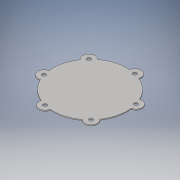
# Autodesk Inventor part: Base_bottom
Saved by Autodesk Inventor 2016 (Build 200138000, 138)
## iProperties
Created: 2015-10-08
Part Number: Base_bottom
Material: Generic
Document SubType Name: Modeling
Designer: powasar16
Density: 1 g/cm^3
Appearance: Default
Author: powasar16
Autodesk Inventor part; units mm, degrees
ref_plane "YZ Plane" through (0, 0, 0) normal (1, 0, 0) x (0, 1, 0)
ref_plane "XZ Plane" through (0, 0, 0) normal (0, 1, 0) x (-1, 0, 0)
ref_plane "XY Plane" through (0, 0, 0) normal (0, 0, 1) x (1, 0, 0)
sketch "Sketch1" plane through (0, 0, 0) normal (0, 1, 0) x (-1, 0, 0)
  circle A0 centre (54.9831, -52.757) radius 12.7
  circle A1 centre (73.1804, 21.2382) radius 12.7
  circle A2 centre (18.1974, 73.9952) radius 12.7
  circle A3 centre (-54.9831, 52.757) radius 12.7
  circle A4 centre (-73.1804, -21.2382) radius 12.7
  circle A5 centre (-18.1974, -73.9952) radius 12.7
  circle A6 centre (54.9831, -52.757) radius 3.75
  circle A7 centre (73.1804, 21.2382) radius 3.75
  circle A8 centre (18.1974, 73.9952) radius 3.75
  circle A9 centre (-54.9831, 52.757) radius 3.75
  circle A10 centre (-73.1804, -21.2382) radius 3.75
  circle A11 centre (-18.1974, -73.9952) radius 3.75
  arc A12 (72.047, 24.8128) -> (21.8158, 73.0104) centre (0, 0) ccw
  arc A13 (57.512, -49.9881) -> (74.1367, 17.6122) centre (0, 0) ccw
  arc A14 (-14.535, -74.8009) -> (52.321, -55.3982) centre (0, 0) ccw
  arc A15 (-72.047, -24.8128) -> (-21.8158, -73.0104) centre (0, 0) ccw
  arc A16 (14.535, 74.8009) -> (-52.321, 55.3982) centre (0, 0) ccw
  arc A17 (-57.512, 49.9881) -> (-74.1367, -17.6122) centre (0, 0) ccw
  point P0 (73.9952, -18.1974)
  dimension "d7" = 25.4
  dimension "d12" = 360
  dimension "d15" = 7.5
  dimension "d18" = 360
  constraints: 25 point on circle, 18 centre point, 2 coincident, 32 other
  measures "d7" diameter of A0
  measures "d15" diameter of A6
extrude "Extrusion1" add sketch "Sketch1" along normal blind 1.905 contours A0 A14 A6 A13 | A13 A6 A14 A0 | A0 A14 A5 A15 A4 A17 A3 A16 A2 A12 A1 A13 | A13 A7 A12 A1 | A1 A12 A7 A13 | A14 A11 A15 A5 | A5 A15 A11 A14 | A12 A8 A16 A2 | A2 A16 A8 A12 | A15 A10 A17 A4 | A4 A17 A10 A15 | A16 A9 A17 A3 | A3 A17 A9 A16
body "Solid1"
